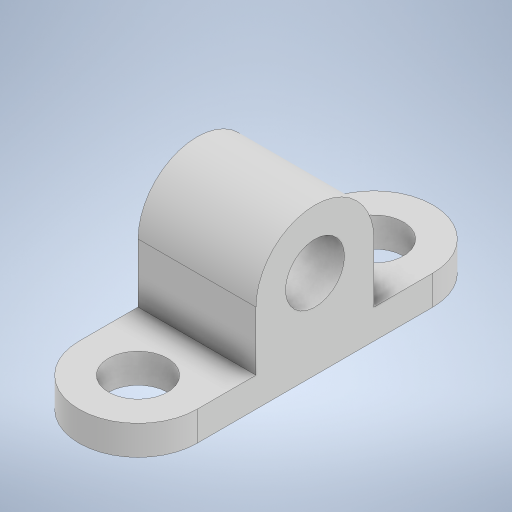
# Autodesk Inventor part: Actividad #1
Saved by Autodesk Inventor 2024 (Build 280153000, 153)
## iProperties
Created: 2024-02-07
Part Number: Actividad #1
Material: Generic
Document SubType Name: Modeling
Designer: benja
Density: 1 g/cm^3
Appearance: Default
Author: benja
Autodesk Inventor part; units mm, degrees
ref_plane "YZ Plane" through (0, 0, 0) normal (1, 0, 0) x (0, 1, 0)
ref_plane "XZ Plane" through (0, 0, 0) normal (0, 1, 0) x (-1, 0, 0)
ref_plane "XY Plane" through (0, 0, 0) normal (0, 0, 1) x (1, 0, 0)
sketch "Sketch1" plane through (0, 0, 0) normal (0, 1, 0) x (-1, 0, 0)
  line L0 (-20, 20) -> (-20, -20)
  line L1 (20, -20) -> (20, 20)
  circle A0 centre (0, 40) radius 10
  arc A1 (20, 40) -> (-20, 40) centre (0, 40) ccw
  circle A2 centre (0, -40) radius 10
  arc A3 (-20, -40) -> (20, -40) centre (0, -40) ccw
  line L2 (20, 20) -> (20, 40)
  line L3 (20, -20) -> (20, -40)
  line L4 (-20, 20) -> (-20, 40)
  line L5 (-20, -20) -> (-20, -40)
  point P0 (0, 0)
  dimension "d0" = 40
  dimension "d1" = 40
  dimension "d3" = 20
  dimension "d4" = 40
  dimension "d6" = 20
  dimension "d7" = 40
  constraints: 12 end point, 4 centre point, 4 point on circle, 2 coincident, 1 parallel, 1 tangent, 1 vertical
  measures "d0" distance of L0.start L0.end
  measures "d1" distance of L1.start L0.end
  measures "d3" diameter of A0
  measures "d4" diameter of A1
  measures "d6" diameter of A2
  measures "d7" diameter of A3
extrude "Extrusion1" add sketch "Sketch1" along normal blind 10
sketch "Sketch2" plane through (20, 0, 40) normal (1, 0, 0) x (0, 0, -1)
  line L0 (80, 10) -> (0, 10) construction
  arc A0 (60, 30) -> (20, 30) centre (40, 30) ccw
  circle A1 centre (40, 30) radius 10
  line L1 (20, 30) -> (20, 10)
  line L2 (60, 30) -> (60, 10)
  line L3 (20, 10) -> (60, 10)
  point P0 (40, 0)
  dimension "d11" = 40
  dimension "d12" = 20
  constraints: 6 end point, 2 centre point, 2 perpendicular, 2 point on circle, 2 point on line, 2 tangent, 1 coincident, 1 collinear
  measures "d11" diameter of A0
  measures "d12" diameter of A1
extrude "Extrusion2" add sketch "Sketch2" against normal blind 40
body "Solid1"
